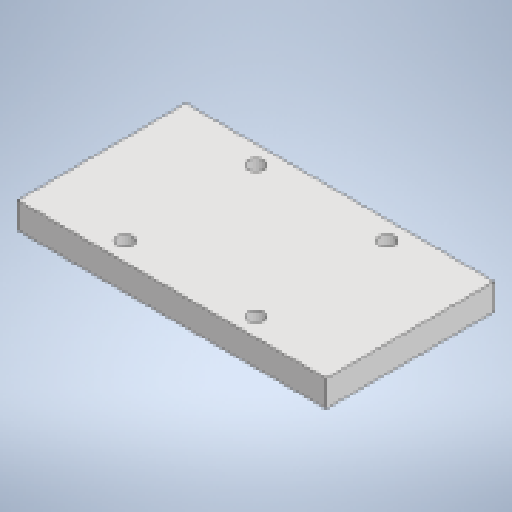
# Autodesk Inventor part: X_Axis_Connector
Saved by Autodesk Inventor 2023 (Build 270158000, 158)
## iProperties
Created: 2022-04-30
Part Number: X_Axis_Connector
Material: Generic
Document SubType Name: Modeling
Designer: plebbb
Density: 1 g/cm^3
Appearance: Default
Author: plebbb
Autodesk Inventor part; units mm, degrees
ref_plane "YZ Plane" through (0, 0, 0) normal (1, 0, 0) x (0, 1, 0)
ref_plane "XZ Plane" through (0, 0, 0) normal (0, 1, 0) x (-1, 0, 0)
ref_plane "XY Plane" through (0, 0, 0) normal (0, 0, 1) x (1, 0, 0)
sketch "Sketch1" plane through (0, 0, 0) normal (0, 1, 0) x (-1, 0, 0)
  line L0 (58.8, 0) -> (0, 0)
  line L1 (0, 0) -> (0, -32)
  line L2 (0, -32) -> (58.8, -32)
  line L3 (58.8, -32) -> (58.8, 0)
  line L4 (41.9, -3.5) -> (16.9, -3.5) construction
  line L5 (16.9, -3.5) -> (16.9, -28.5) construction
  line L6 (16.9, -28.5) -> (41.9, -28.5) construction
  line L7 (41.9, -28.5) -> (41.9, -3.5) construction
  circle A0 centre (41.9, -3.5) radius 1.5
  circle A1 centre (16.9, -3.5) radius 1.5
  circle A2 centre (41.9, -28.5) radius 1.5
  circle A3 centre (16.9, -28.5) radius 1.5
  point P0 (41.9, -16)
  point P1 (58.8, -16)
  point P2 (29.4, -28.5)
  point P3 (29.4, -32)
  dimension "d0" = 3
  dimension "d1" = 25
  dimension "d2" = 32
  dimension "d3" = 58.8
  constraints: 16 end point, 5 coincident, 4 centre point, 4 midpoint, 4 parallel, 3 equal radius, 3 perpendicular, 2 horizontal, 1 horizontal alignment, 1 vertical alignment
  measures "d0" diameter of A0
  measures "d1" distance of L6.end L4.start
  measures "d2" distance of L2.end L0.start
  measures "d3" distance of L1.end L2.end
extrude "Extrusion1" add sketch "Sketch1" along normal blind 2
sketch "Sketch2" plane through (-58.8, 0, -32) normal (-1, 0, 0) x (0, 0, 1)
  circle A0 centre (31, 17.2) radius 16 construction
  circle A1 centre (42.3137, 28.5137) radius 2.4
  circle A2 centre (15, 17.2) radius 2.4
  circle A3 centre (19.6863, 5.8863) radius 2.4
  circle A4 centre (19.6863, 28.5137) radius 2.4
  circle A5 centre (47, 17.2) radius 2.4
  circle A6 centre (42.3137, 5.8863) radius 2.4
  line L0 (19.6863, 28.5137) -> (42.3137, 5.8863) construction
  line L1 (15, 17.2) -> (31, 17.2) construction
  line L2 (0, 2) -> (32, 2) projected
  arc A7 (43.0482, 0) -> (16.51, 2) centre (31, 17.2) ccw
  line L3 (0, 0) -> (32, 0) projected
  line L4 (32, 0) -> (43.0482, 0)
  line L5 (32, 0) -> (32, 2) projected
  line L6 (0, 2) -> (0, 38.2)
  line L7 (0, 38.2) -> (31, 38.2)
  circle A8 centre (31, 17.2) radius 6.25
  point P0 (31, 17.2)
  dimension "d6" = 4.8
  dimension "d7" = 32
  dimension "d9" = 15.2
  dimension "d11" = 45
  dimension "d12" = 31
  dimension "d14" = 21
  dimension "d17" = 12.5
  constraints: 10 end point, 9 centre point, 9 point on circle, 5 equal radius, 2 coincident, 2 horizontal alignment, 2 midpoint, 2 perpendicular, 2 vertical alignment, 1 point on line, 1 tangent, 1 vertical
  measures "d6" diameter of A1
  measures "d7" diameter of A0
  measures "d9" vertical distance of L2.start L1.end
  measures "d11" angle of L0 L1
  measures "d12" horizontal distance of L2.start L1.end
  measures "d14" radius of A7
  measures "d17" diameter of A8
extrude "Extrusion2" add sketch "Sketch2" against normal up to surface (58.8 mm away)
sketch "Sketch3" plane through (-58.8, 0, -32) normal (-1, 0, 0) x (0, 0, 1)
  circle A0 centre (31, 17.2) radius 10.025
  circle A1 centre (31, 17.2) radius 6.25 construction
  point P0 (32, 0)
  dimension "d18" = 20.05
  constraints: 1 centre point, 1 concentric
  measures "d18" diameter of A0
extrude "Extrusion3" cut sketch "Sketch3" against normal blind 27.05
sketch "Sketch4" plane through (-58.8, 38.2, -1) normal (0, 1, 0) x (1, 0, 0)
  circle A0 centre (41.9, 2.5) radius 1.5 projected
  circle A1 centre (41.9, 27.5) radius 1.5 projected
  circle A2 centre (16.9, 2.5) radius 1.5 projected
  circle A3 centre (16.9, 27.5) radius 1.5 projected
  circle A4 centre (16.9, 2.5) radius 3
  circle A5 centre (16.9, 27.5) radius 3
  circle A6 centre (41.9, 27.5) radius 3
  circle A7 centre (41.9, 2.5) radius 3
  point P0 (58.8, -1)
  dimension "d21" = 6
  constraints: 4 centre point, 4 concentric, 3 equal radius
  measures "d21" diameter of A6
extrude "Extrusion4" cut sketch "Sketch4" against normal up to surface (36.2 mm away) contours A0 | A1 | A2 | A3 | A4 | A5 | A6 | A7
body "Solid1"
